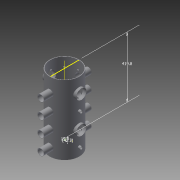
# Autodesk Inventor part: Detection Region Vacuum Collar v2
Saved by Autodesk Inventor 2015 (Build 190159000, 159)
## iProperties
Created: 2014-06-20
Part Number: Detection Region Vacuum Collar v2
Material: Generic
Document SubType Name: Modeling
Designer: Aki
Density: 1 g/cm^3
Appearance: Default
Author: Aki
Autodesk Inventor part; units mm, degrees
sketch "Sketch1" plane through (0, 0, 0) normal (0, 1, 0) x (-1, 0, 0)
  circle A0 centre (0, 0) radius 101.6
  circle A1 centre (0, 0) radius 97.6
  dimension "d0" = 203.2
  dimension "d3" = 195.2
  constraints: 2 centre point, 2 coincident
  measures "d0" diameter of A0
  measures "d3" diameter of A1
extrude "Extrusion2" add sketch "Sketch1" along normal blind 477.1
ref_plane "Work Plane1" through (0, 0, 101.6) normal (0, 0, 1) x (1, 0, 0)
sketch "Sketch2" plane through (0, 0, 101.6) normal (0, 0, 1) x (1, 0, 0)
  circle A0 centre (0, 57.3) radius 22.25
  circle A1 centre (0, 164.8) radius 22.25
  circle A2 centre (0, 272.3) radius 22.25
  circle A3 centre (0, 379.8) radius 22.25
  line L0 (101.6, 477.1) -> (-101.6, 477.1) projected
  line L1 (-101.6, 0) -> (101.6, 0) projected
  point P0 (0, 0)
  dimension "d7" = 44.5
  dimension "d8" = 44.5
  dimension "d9" = 44.5
  dimension "d10" = 44.5
  dimension "d11" = 97.3
  dimension "d12" = 57.3
  dimension "d13" = 215
  dimension "d14" = 215
  constraints: 4 centre point
  measures "d7" diameter of A0
  measures "d8" diameter of A1
  measures "d9" diameter of A2
  measures "d10" diameter of A3
  measures "d11" distance from line of L0 A3.centre
  measures "d12" distance from line of L1 A0.centre
  measures "d13" distance of A2.centre A0.centre
  measures "d14" distance of A3.centre A1.centre
extrude "Extrusion8" add sketch "Sketch2" against normal up to next
sketch "Sketch13" plane through (0, 0, 101.6) normal (0, 0, 1) x (1, 0, 0)
  circle A0 centre (0, 57.3) radius 22.25
  circle A1 centre (0, 164.8) radius 22.25
  circle A2 centre (0, 272.3) radius 22.25
  circle A3 centre (0, 379.8) radius 22.25
  line L0 (101.6, 477.1) -> (-101.6, 477.1) projected
  line L1 (-101.6, 0) -> (101.6, 0) projected
  point P0 (0, 0)
  dimension "d104" = 44.5
  dimension "d105" = 44.5
  dimension "d106" = 44.5
  dimension "d107" = 44.5
  dimension "d108" = 97.3
  dimension "d109" = 57.3
  dimension "d110" = 215
  dimension "d111" = 215
  constraints: 4 centre point
  measures "d104" diameter of A0
  measures "d105" diameter of A1
  measures "d106" diameter of A2
  measures "d107" diameter of A3
  measures "d108" distance from line of L0 A3.centre
  measures "d109" distance from line of L1 A0.centre
  measures "d110" distance of A2.centre A0.centre
  measures "d111" distance of A3.centre A1.centre
extrude "Extrusion9" add sketch "Sketch13" along normal blind 62.5
ref_plane "Work Plane2" through (0, 0, -101.6) normal (0, 0, 1) x (1, 0, 0)
sketch "Sketch3" plane through (0, 0, -101.6) normal (0, 0, 1) x (1, 0, 0)
  circle A0 centre (0, 57.3) radius 22.25
  circle A1 centre (0, 164.8) radius 22.25
  circle A2 centre (0, 272.3) radius 22.25
  circle A3 centre (0, 379.8) radius 22.25
  line L0 (101.6, 477.1) -> (-101.6, 477.1) projected
  line L1 (-101.6, 0) -> (101.6, 0) projected
  line L2 (0, 357.55) -> (0, 402.05) projected
  point P0 (0, 0)
  dimension "d18" = 44.5
  dimension "d19" = 44.5
  dimension "d20" = 44.5
  dimension "d21" = 44.5
  dimension "d22" = 97.3
  dimension "d23" = 57.3
  dimension "d24" = 215
  dimension "d25" = 215
  dimension "d26" = 0
  constraints: 4 centre point
  measures "d18" diameter of A0
  measures "d19" diameter of A1
  measures "d20" diameter of A2
  measures "d21" diameter of A3
  measures "d22" distance from line of L0 A3.centre
  measures "d23" distance from line of L1 A0.centre
  measures "d24" distance of A0.centre A2.centre
  measures "d25" distance of A3.centre A1.centre
  measures "d26" distance from line of L2 A3.centre
extrude "Extrusion10" add sketch "Sketch3" along normal up to next
sketch "Sketch14" plane through (0, 0, -101.6) normal (0, 0, 1) x (1, 0, 0)
  circle A0 centre (0, 57.3) radius 22.25
  circle A1 centre (0, 164.8) radius 22.25 projected
  circle A2 centre (0, 164.8) radius 22.25
  circle A3 centre (0, 272.3) radius 22.25
  circle A4 centre (0, 379.8) radius 22.25
  line L0 (-101.6, 0) -> (101.6, 0) projected
  line L1 (101.6, 477.1) -> (-101.6, 477.1) projected
  point P0 (0, 0)
  dimension "d116" = 44.5
  dimension "d117" = 44.5
  dimension "d118" = 44.5
  dimension "d119" = 44.5
  dimension "d120" = 57.3
  dimension "d121" = 215
  dimension "d122" = 215
  dimension "d123" = 97.3
  constraints: 4 centre point, 1 coincident
  measures "d116" diameter of A0
  measures "d117" diameter of A2
  measures "d118" diameter of A3
  measures "d119" diameter of A4
  measures "d120" distance from line of L0 A0.centre
  measures "d121" distance of A3.centre A0.centre
  measures "d122" distance of A4.centre A2.centre
  measures "d123" distance from line of L1 A4.centre
extrude "Extrusion11" add sketch "Sketch14" against normal blind 62.5
sketch "Sketch15" plane through (0, 379.8, -164.1) normal (0, 0, -1) x (-1, 0, 0)
  circle A0 centre (0, -322.5106) radius 21.35
  point P0 (0, -379.8)
  dimension "d126" = 42.7
  constraints: 1 centre point
  measures "d126" diameter of A0
hole "Hole8" at (0, 57.2894, -164.1) direction (0, 0, 1) diameter 42.7 end through all
sketch "Sketch16" plane through (0, 164.8, -164.1) normal (0, 0, -1) x (-1, 0, 0)
  circle A0 centre (0, 0) radius 21.35
  point P0 (0, -164.8)
  dimension "d134" = 42.7
  constraints: 1 centre point
  measures "d134" diameter of A0
hole "Hole9" at (0, 164.8, -164.1) direction (0, 0, 1) diameter 42.7 end through all
sketch "Sketch17" plane through (0, 272.3, -164.1) normal (0, 0, -1) x (-1, 0, 0)
  circle A0 centre (0, 0) radius 21.35
  point P0 (0, -272.3)
  dimension "d142" = 42.7
  constraints: 1 centre point
  measures "d142" diameter of A0
hole "Hole10" at (0, 272.3, -164.1) direction (0, 0, 1) diameter 42.7 end through all
sketch "Sketch18" plane through (0, 379.8, -164.1) normal (0, 0, -1) x (-1, 0, 0)
  circle A0 centre (0, 0) radius 21.35
  point P0 (0, -379.8)
  dimension "d150" = 42.7
  constraints: 1 centre point
  measures "d150" diameter of A0
hole "Hole11" at (0, 379.8, -164.1) direction (0, 0, 1) diameter 42.7 end through all
ref_plane "Work Plane3" through (101.6, 0, 0) normal (1, 0, 0) x (0, 1, 0)
sketch "Sketch27" plane through (101.6, 0, 0) normal (1, 0, 0) x (0, 1, 0)
  circle A0 centre (164.8, 0) radius 35.05
  circle A1 centre (379.8, 0) radius 35.05
  line L0 (477.1, -101.6) -> (477.1, 101.6) projected
  circle A2 centre (272.3, 0) radius 9.65
  circle A3 centre (57.3, 0) radius 9.65
  point P0 (0, 0)
  dimension "d204" = 70.1
  dimension "d205" = 70.1
  dimension "d206" = 97.3
  dimension "d207" = 215
  dimension "d208" = 19.3
  dimension "d209" = 19.3
  dimension "d210" = 215
  dimension "d211" = 107.5
  constraints: 4 centre point
  measures "d204" diameter of A0
  measures "d205" diameter of A1
  measures "d206" distance from line of L0 A1.centre
  measures "d207" distance of A0.centre A1.centre
  measures "d208" diameter of A2
  measures "d209" diameter of A3
  measures "d210" distance of A3.centre A2.centre
  measures "d211" distance of A2.centre A1.centre
extrude "Extrusion17" add sketch "Sketch27" against normal up to next
sketch "Sketch28" plane through (101.6, 0, 0) normal (1, 0, 0) x (0, 1, 0)
  circle A0 centre (57.3, 0) radius 9.65
  circle A1 centre (272.3, 0) radius 9.65
  circle A2 centre (164.8, 0) radius 35.05
  circle A3 centre (379.8, 0) radius 35.05
  line L0 (477.1, -101.6) -> (477.1, 101.6) projected
  point P0 (0, 0)
  dimension "d214" = 19.3
  dimension "d215" = 19.3
  dimension "d216" = 70.1
  dimension "d217" = 70.1
  dimension "d218" = 97.3
  dimension "d219" = 107.5
  dimension "d220" = 215
  dimension "d221" = 215
  constraints: 4 centre point
  measures "d214" diameter of A0
  measures "d215" diameter of A1
  measures "d216" diameter of A2
  measures "d217" diameter of A3
  measures "d218" distance from line of L0 A3.centre
  measures "d219" distance of A1.centre A3.centre
  measures "d220" distance of A2.centre A3.centre
  measures "d221" distance of A1.centre A0.centre
extrude "Extrusion18" add sketch "Sketch28" along normal blind 15
ref_plane "Work Plane8" through (-101.6, 0, 0) normal (1, 0, 0) x (0, 1, 0)
sketch "Sketch33" plane through (-101.6, 0, 0) normal (1, 0, 0) x (0, 1, 0)
  circle A0 centre (164.8, 0) radius 35.05
  circle A1 centre (379.8, 0) radius 35.05
  line L0 (477.1, -101.6) -> (477.1, 101.6) projected
  circle A2 centre (272.3, 0) radius 9.515
  circle A3 centre (57.3, 0) radius 9.65 projected
  circle A4 centre (57.3, 0) radius 9.65
  point P0 (0, 0)
  dimension "d230" = 70.1
  dimension "d231" = 70.1
  dimension "d232" = 97.3
  dimension "d233" = 215
  dimension "d234" = 19.03
  dimension "d235" = 107.5
  dimension "d236" = 19.3
  dimension "d237" = 215
  constraints: 4 centre point, 1 coincident
  measures "d230" diameter of A0
  measures "d231" diameter of A1
  measures "d232" distance from line of L0 A1.centre
  measures "d233" distance of A0.centre A1.centre
  measures "d234" diameter of A2
  measures "d235" distance of A1.centre A2.centre
  measures "d236" diameter of A4
  measures "d237" distance of A2.centre A4.centre
extrude "Extrusion19" add sketch "Sketch33" along normal up to next
sketch "Sketch34" plane through (-101.6, 0, 0) normal (1, 0, 0) x (0, 1, 0)
  circle A0 centre (379.8, 0) radius 35.05
  circle A1 centre (164.8, 0) radius 35.05
  line L0 (477.1, -101.6) -> (477.1, 101.6) projected
  arc A2 (262.785, 0) -> (281.815, 0) centre (272.3, 0) ccw projected
  circle A3 centre (272.3, 0) radius 9.65
  arc A4 (66.95, 0) -> (47.65, 0) centre (57.3, 0) ccw projected
  circle A5 centre (57.3, 0) radius 9.65
  point P0 (0, 0)
  point P1 (312.785, 0)
  point P2 (331.815, 0)
  point P3 (97.65, 0)
  point P4 (116.95, 0)
  point P5 (252.785, 0)
  point P6 (271.815, 0)
  point P7 (37.65, 0)
  point P8 (56.95, 0)
  dimension "d240" = 70.1
  dimension "d241" = 70.1
  dimension "d242" = 97.3
  dimension "d243" = 215
  dimension "d244" = 19.3
  dimension "d245" = 19.3
  dimension "d246" = 107.5
  dimension "d247" = 215
  constraints: 4 centre point, 2 coincident, 2 other
  measures "d240" diameter of A0
  measures "d241" diameter of A1
  measures "d242" distance from line of L0 A0.centre
  measures "d243" distance of A1.centre A0.centre
  measures "d244" diameter of A3
  measures "d245" diameter of A5
  measures "d246" distance of A3.centre A0.centre
  measures "d247" distance of A5.centre A3.centre
extrude "Extrusion20" add sketch "Sketch34" against normal blind 15
sketch "Sketch29" plane through (116.6, 379.8, 0) normal (1, 0, 0) x (0, 0, -1)
  circle A0 centre (0, 0) radius 34.15
  line L0 (101.6, 97.3) -> (-101.6, 97.3) projected
  point P0 (0, -379.8)
  dimension "d224" = 68.3
  dimension "d225" = 97.3
  constraints: 1 centre point
  measures "d224" diameter of A0
  measures "d225" distance from line of L0 A0.centre
sketch "Sketch30" plane through (116.6, 164.8, 0) normal (1, 0, 0) x (0, 0, -1)
  circle A0 centre (0, 0) radius 34.15
  point P0 (0, -164.8)
  dimension "d226" = 68.3
  constraints: 1 centre point
  measures "d226" diameter of A0
sketch "Sketch31" plane through (116.6, 272.3, 0) normal (1, 0, 0) x (0, 0, -1)
  circle A0 centre (0, 0) radius 8
  point P0 (0, -272.3)
  dimension "d227" = 16
  constraints: 1 centre point
  measures "d227" diameter of A0
sketch "Sketch32" plane through (116.6, 57.3, 0) normal (1, 0, 0) x (0, 0, -1)
  circle A0 centre (0, 0) radius 8
  point P0 (0, -57.3)
  dimension "d228" = 16
  constraints: 1 centre point
  measures "d228" diameter of A0
hole "Hole15" at (116.6, 379.8, 0) direction (-1, 0, 0) diameter 68.3 end through all
hole "Hole16" at (116.6, 164.8, 0) direction (-1, 0, 0) diameter 68.3 end through all
hole "Hole17" at (116.6, 272.3, 0) direction (-1, 0, 0) diameter 16 end through all
hole "Hole18" at (116.6, 57.3, 0) direction (-1, 0, 0) diameter 16 end through all
ref_plane "Work Plane9" through (0, 10, 0) normal (0, 1, 0) x (-1, 0, 0)
sketch "Sketch36" plane through (0, 10, 0) normal (0, 1, 0) x (-1, 0, 0)
  circle A0 centre (0, 0) radius 97.6
  circle A1 centre (0, 0) radius 88.6
  dimension "d283" = 195.2
  dimension "d284" = 177.2
  constraints: 2 centre point, 2 coincident
  measures "d283" diameter of A0
  measures "d284" diameter of A1
extrude "Extrusion22" add sketch "Sketch36" along normal blind 5
sketch "Sketch37" plane through (0, 15, 0) normal (0, 1, 0) x (1, 0, 0)
  circle A0 centre (0, 0) radius 91.55 construction
  circle A1 centre (0, 91.55) radius 2.15
  circle A2 centre (-91.55, 0) radius 2.15
  circle A3 centre (91.55, 0) radius 2.15
  circle A4 centre (0, -91.55) radius 2.15
  circle A5 centre (-64.7356, 64.7356) radius 2.15
  circle A6 centre (64.7356, 64.7356) radius 2.15
  circle A7 centre (-64.7356, -64.7356) radius 2.15
  circle A8 centre (64.7356, -64.7356) radius 2.15
  dimension "d287" = 183.1
  dimension "d288" = 4.3
  dimension "d289" = 4.3
  dimension "d290" = 4.3
  dimension "d291" = 4.3
  dimension "d292" = 4.3
  dimension "d293" = 4.3
  dimension "d294" = 4.3
  dimension "d295" = 4.3
  dimension "d296" = 45
  dimension "d297" = 45
  dimension "d298" = 0
  dimension "d299" = 90
  dimension "d300" = 45
  dimension "d301" = 90
  dimension "d302" = 45
  dimension "d303" = 90
  constraints: 8 centre point, 1 coincident, 10 other
  measures "d288" diameter of A1
  measures "d289" diameter of A2
  measures "d290" diameter of A3
  measures "d291" diameter of A4
  measures "d292" diameter of A5
  measures "d293" diameter of A6
  measures "d294" diameter of A7
  measures "d295" diameter of A8
  measures "d298" vertical distance of point (0, 0) A2.centre
extrude "Extrusion23" cut sketch "Sketch37" against normal blind 6
thread "Thread1" size "M4.5x0.75" class "6H" standard "ANSI Metric M Profile" full length
thread "Thread2" size "M4.5x0.75" class "6H" standard "ANSI Metric M Profile" full length
thread "Thread3" size "M4.5x0.75" class "6H" standard "ANSI Metric M Profile" full length
thread "Thread4" size "M4.5x0.75" class "6H" standard "ANSI Metric M Profile" full length
thread "Thread5" size "M4.5x0.75" class "6H" standard "ANSI Metric M Profile" full length
thread "Thread6" size "M4.5x0.75" class "6H" standard "ANSI Metric M Profile" full length
thread "Thread7" size "M4.5x0.75" class "6H" standard "ANSI Metric M Profile" full length
thread "Thread8" size "M4.5x0.75" class "6H" standard "ANSI Metric M Profile" full length
thread "Thread9" size "M4.5x0.75" class "6H" standard "ANSI Metric M Profile" full length
sketch "Sketch38" plane through (0, 0, 0) normal (1, 0, 0) x (0, 1, 0)
  circle A0 centre (57.3, 0) radius 9.65
  line L0 (477.1, 97.6) -> (477.1, -97.6) projected
  line L1 (15, 88.6) -> (15, -88.6) projected
  point P0 (0, 0)
  dimension "d324" = 19.3
  dimension "d325" = 419.8
  dimension "d326" = 42.3
  constraints: 1 centre point
  measures "d324" diameter of A0
  measures "d325" distance from line of L0 A0.centre
  measures "d326" distance from line of L1 A0.centre
ref_plane "Work Plane10" through (0, 415.3, 0) normal (0, 1, 0) x (-1, 0, 0)
sketch "Sketch39" plane through (0, 415.3, 0) normal (0, 1, 0) x (-1, 0, 0)
  line L0 (-5, 106.5332) -> (-5, 88.5332)
  line L1 (-5, 88.5332) -> (5, 88.5332)
  line L2 (5, 88.5332) -> (5, 106.5332)
  line L3 (5, 106.5332) -> (-5, 106.5332)
  line L4 (-5, 106.5332) -> (5, 88.5332) construction
  line L5 (-5, 88.5332) -> (5, 106.5332) construction
  line L6 (-5, 106.5332) -> (13, 106.5332) construction
  line L7 (-79.1781, 71.576) -> (-66.4502, 58.8481)
  line L8 (-66.4502, 58.8481) -> (-59.3791, 65.9192)
  line L9 (-59.3791, 65.9192) -> (-72.1071, 78.6471)
  line L10 (-72.1071, 78.6471) -> (-79.1781, 71.576)
  line L11 (-79.1781, 71.576) -> (-59.3791, 65.9192) construction
  line L12 (-66.4502, 58.8481) -> (-72.1071, 78.6471) construction
  line L13 (-79.1781, 71.576) -> (-61.1781, 71.576) construction
  line L14 (72.1071, 78.6471) -> (59.3791, 65.9192)
  line L15 (59.3791, 65.9192) -> (66.4502, 58.8481)
  line L16 (66.4502, 58.8481) -> (79.1781, 71.576)
  line L17 (79.1781, 71.576) -> (72.1071, 78.6471)
  line L18 (72.1071, 78.6471) -> (66.4502, 58.8481) construction
  line L19 (59.3791, 65.9192) -> (79.1781, 71.576) construction
  line L20 (72.1071, 78.6471) -> (90.1071, 78.6471) construction
  line L21 (-106.6, -5) -> (-88.6, -5)
  line L22 (-88.6, -5) -> (-88.6, 5)
  line L23 (-88.6, 5) -> (-106.6, 5)
  line L24 (-106.6, 5) -> (-106.6, -5)
  line L25 (-106.6, -5) -> (-88.6, 5) construction
  line L26 (-88.6, -5) -> (-106.6, 5) construction
  line L27 (-106.6, -5) -> (-88.6, -5) construction
  line L28 (106.6, -5) -> (88.6, -5)
  line L29 (88.6, -5) -> (88.6, 5)
  line L30 (88.6, 5) -> (106.6, 5)
  line L31 (106.6, 5) -> (106.6, -5)
  line L32 (106.6, -5) -> (88.6, 5) construction
  line L33 (88.6, -5) -> (106.6, 5) construction
  line L34 (106.6, -5) -> (124.6, -5) construction
  line L35 (79.1781, -71.576) -> (66.4502, -58.8481)
  line L36 (66.4502, -58.8481) -> (59.3791, -65.9192)
  line L37 (59.3791, -65.9192) -> (72.1071, -78.6471)
  line L38 (72.1071, -78.6471) -> (79.1781, -71.576)
  line L39 (79.1781, -71.576) -> (59.3791, -65.9192) construction
  line L40 (66.4502, -58.8481) -> (72.1071, -78.6471) construction
  line L41 (79.1781, -71.576) -> (97.1781, -71.576) construction
  line L42 (-5, -106.6) -> (-5, -88.6)
  line L43 (-5, -88.6) -> (5, -88.6)
  line L44 (5, -88.6) -> (5, -106.6)
  line L45 (5, -106.6) -> (-5, -106.6)
  line L46 (-5, -106.6) -> (5, -88.6) construction
  line L47 (-5, -88.6) -> (5, -106.6) construction
  line L48 (-5, -106.6) -> (13, -106.6) construction
  line L49 (-79.1781, -71.576) -> (-66.4502, -58.8481)
  line L50 (-66.4502, -58.8481) -> (-59.3791, -65.9192)
  line L51 (-59.3791, -65.9192) -> (-72.1071, -78.6471)
  line L52 (-72.1071, -78.6471) -> (-79.1781, -71.576)
  line L53 (-79.1781, -71.576) -> (-59.3791, -65.9192) construction
  line L54 (-66.4502, -58.8481) -> (-72.1071, -78.6471) construction
  line L55 (-79.1781, -71.576) -> (-61.1781, -71.576) construction
  circle A0 centre (0, 0) radius 97.6
  point P0 (0, 97.5332)
  point P1 (-69.2786, 68.7476)
  point P2 (69.2786, 68.7476)
  point P3 (-97.6, 0)
  point P4 (97.6, 0)
  point P5 (69.2786, -68.7476)
  point P6 (0, -97.6)
  point P7 (-69.2786, -68.7476)
  dimension "d331" = 18
  dimension "d332" = 90
  dimension "d333" = 10
  dimension "d334" = 18
  dimension "d335" = 45
  dimension "d336" = 10
  dimension "d337" = 18
  dimension "d338" = 135
  dimension "d339" = 10
  dimension "d340" = 18
  dimension "d341" = 0
  dimension "d342" = 10
  dimension "d343" = 18
  dimension "d344" = 180
  dimension "d345" = 10
  dimension "d346" = 18
  dimension "d347" = 135
  dimension "d348" = 10
  dimension "d349" = 18
  dimension "d350" = 90
  dimension "d351" = 10
  dimension "d352" = 18
  dimension "d353" = 45
  dimension "d354" = 10
  dimension "d356" = 195.2
  constraints: 112 end point, 21 parallel, 16 midpoint, 8 equal length, 8 horizontal, 8 perpendicular, 1 centre point, 1 coincident, 1 collinear, 1 vertical
  measures "d331" distance of L0.start L0.end
  measures "d332" angle of L0 L6
  measures "d333" distance of L1.end L0.end
  measures "d334" distance of L7.start L7.end
  measures "d335" angle of L7 L13
  measures "d336" distance of L8.end L7.end
  measures "d337" distance of L14.start L14.end
  measures "d338" angle of L14 L20
  measures "d339" distance of L15.end L14.end
  measures "d340" distance of L21.start L21.end
  measures "d341" distance between parallel lines of L21 L27
  measures "d342" distance of L22.end L21.end
  measures "d343" distance of L28.start L28.end
  measures "d344" angle of L28 L34
  measures "d345" distance of L28.end L29.end
  measures "d346" distance of L35.start L35.end
  measures "d347" angle of L41 L35
  measures "d348" distance of L36.end L35.end
  measures "d349" distance of L42.start L42.end
  measures "d350" angle of L48 L42
  measures "d351" distance of L42.end L43.end
  measures "d352" distance of L49.start L49.end
  measures "d353" angle of L55 L49
  measures "d354" distance of L49.end L50.end
  measures "d356" diameter of A0
extrude "Extrusion24" add sketch "Sketch39" along normal blind 4 contours L3 L2 A0 L0 | A0 L2 L1 L0 | A0 L7 L10 L9 | L9 L8 L7 A0 | A0 L16 L15 L14 | L14 L17 L16 A0 | A0 L21 L24 L23 | L23 L22 L21 A0 | A0 L28 L29 L30 | L30 L31 L28 A0 | A0 L51 L52 L49 | L49 L50 L51 A0 | A0 L37 L36 L35 | L35 L38 L37 A0 | A0 L44 L45 L42 | L42 L43 L44 A0
sketch "Sketch40" plane through (0, 415.3, 0) normal (0, 1, 0) x (-1, 0, 0)
  circle A0 centre (0, 0) radius 101.6
  circle A1 centre (0, 0) radius 111.8636
  dimension "d359" = 203.2
  constraints: 2 centre point, 2 coincident
  measures "d359" diameter of A0
extrude "Extrusion25" cut sketch "Sketch40" along normal blind 5
sketch "Sketch41" plane through (0, 419.3, 0) normal (0, 1, 0) x (1, 0, 0)
  circle A0 centre (-65.0006, 64.4696) radius 2.15
  line L0 (-59.3791, 65.9192) -> (-65.6661, 72.2061) projected
  point P0 (0, 0)
  dimension "d362" = 4.3
  dimension "d363" = 91.55
  dimension "d364" = 5
  constraints: 1 centre point
  measures "d362" diameter of A0
  measures "d363" distance of point (0, 0) A0.centre
  measures "d364" distance from line of L0 A0.centre
hole "Hole19" at (-65.0006, 419.3, -64.4696) direction (0, -1, 0) diameter 4.3 end through all
sketch "Sketch42" plane through (0, 419.3, 0) normal (0, 1, 0) x (1, 0, 0)
  circle A0 centre (-91.55, 0) radius 2.15
  line L0 (-88.6, 5) -> (-97.4718, 5) projected
  point P0 (0, 0)
  dimension "d372" = 4.3
  dimension "d373" = 91.55
  dimension "d374" = 5
  constraints: 1 centre point
  measures "d372" diameter of A0
  measures "d373" distance of point (0, 0) A0.centre
  measures "d374" distance from line of L0 A0.centre
hole "Hole20" at (-91.55, 419.3, 0) direction (0, -1, 0) diameter 4.3 end through all
sketch "Sketch43" plane through (0, 419.3, 0) normal (0, 1, 0) x (1, 0, 0)
  circle A0 centre (0, 91.55) radius 2.15
  point P0 (0, 0)
  dimension "d382" = 4.3
  dimension "d383" = 91.55
  constraints: 1 centre point
  measures "d382" diameter of A0
  measures "d383" distance of A0.centre point (0, 0)
hole "Hole21" at (0, 419.3, -91.55) direction (0, -1, 0) diameter 4.3 end through all
sketch "Sketch44" plane through (0, 419.3, 0) normal (0, 1, 0) x (1, 0, 0)
  circle A0 centre (65.0006, 64.4696) radius 2.15
  line L0 (65.6661, 72.2061) -> (59.3791, 65.9192) projected
  point P0 (0, 0)
  dimension "d391" = 4.3
  dimension "d392" = 91.55
  dimension "d393" = 5
  constraints: 1 centre point
  measures "d391" diameter of A0
  measures "d392" distance of point (0, 0) A0.centre
  measures "d393" distance from line of L0 A0.centre
hole "Hole22" at (65.0006, 419.3, -64.4696) direction (0, -1, 0) diameter 4.3 end through all
sketch "Sketch45" plane through (0, 419.3, 0) normal (0, 1, 0) x (1, 0, 0)
  circle A0 centre (91.55, 0) radius 2.15 projected
  circle A1 centre (91.55, 0) radius 2.15
  point P0 (0, 0)
  dimension "d401" = 4.3
  dimension "d402" = 91.55
  constraints: 1 centre point, 1 coincident
  measures "d401" diameter of A1
  measures "d402" distance of A1.centre point (0, 0)
hole "Hole23" at (91.55, 419.3, 0) direction (0, -1, 0) diameter 4.3 end through all
sketch "Sketch46" plane through (0, 419.3, 0) normal (0, 1, 0) x (1, 0, 0)
  circle A0 centre (64.7356, -64.7356) radius 2.15 projected
  circle A1 centre (64.7356, -64.7356) radius 2.15
  point P0 (0, 0)
  dimension "d410" = 4.3
  constraints: 1 centre point, 1 coincident
  measures "d410" diameter of A1
hole "Hole24" at (64.7356, 419.3, 64.7356) direction (0, -1, 0) diameter 4.3 end through all
sketch "Sketch47" plane through (0, 419.3, 0) normal (0, 1, 0) x (1, 0, 0)
  circle A0 centre (0, -91.55) radius 2.15
  point P0 (0, 0)
  dimension "d418" = 4.3
  dimension "d419" = 91.55
  constraints: 1 centre point
  measures "d418" diameter of A0
  measures "d419" distance of point (0, 0) A0.centre
hole "Hole25" at (0, 419.3, 91.55) direction (0, -1, 0) diameter 4.3 end through all
sketch "Sketch48" plane through (0, 419.3, 0) normal (0, 1, 0) x (1, 0, 0)
  circle A0 centre (-64.7356, -64.7356) radius 2.15 projected
  circle A1 centre (-64.7356, -64.7356) radius 2.15
  point P0 (0, 0)
  dimension "d427" = 4.3
  constraints: 1 centre point, 1 coincident
  measures "d427" diameter of A1
hole "Hole26" at (-64.7356, 419.3, 64.7356) direction (0, -1, 0) diameter 4.3 end through all
thread "Thread10" size "M4.5x0.75" class "6H" standard "ANSI Metric M Profile" full length
thread "Thread11" size "M4.5x0.75" class "6H" standard "ANSI Metric M Profile" full length
thread "Thread12" size "M4.5x0.75" class "6H" standard "ANSI Metric M Profile" full length
thread "Thread13" size "M4.5x0.75" class "6H" standard "ANSI Metric M Profile" full length
thread "Thread14" size "M4.5x0.75" class "6H" standard "ANSI Metric M Profile" full length
thread "Thread15" size "M4.5x0.75" class "6H" standard "ANSI Metric M Profile" full length
thread "Thread16" size "M4.5x0.75" class "6H" standard "ANSI Metric M Profile" full length
thread "Thread17" size "M4.5x0.75" class "6H" standard "ANSI Metric M Profile" full length
body "Solid2"
